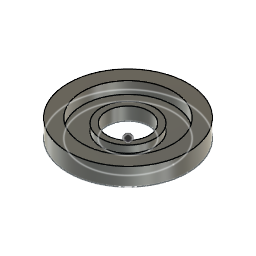
cap modified (Autodesk Fusion 360 design; units mm, degrees)
part number: 2025-11-25-15-10-51-182
Autodesk Fusion 360 part; units mm, degrees
sketch "Sketch1" plane through (0, 0, 0) normal (0, 0, 1) x (1, 0, 0)
  circle A0 centre (0, 0) radius 17.65
  circle A1 centre (0, 0) radius 38
  circle A2 centre (0, 0) radius 50
  dimension "d1" = 35.3
  dimension "d2" = 76
  dimension "d3" = 100
  constraint coincident A0.centre A1.centre
  measures "d1" diameter of A0
  measures "d2" diameter of A1
  measures "d3" diameter of A2
extrude "Extrude1" add sketch "Sketch1" along normal blind 5 contours A1
extrude "Extrude2" add sketch "Sketch1" along normal blind 15 contours A2
sketch "Sketch2" plane through (0, 0, 5) normal (0, 0, 1) x (-1, 0, 0)
  circle A0 centre (0, 0) radius 17.65
  circle A1 centre (0, 0) radius 38
  circle A2 centre (0, 0) radius 22.5
  dimension "d8" = 45
  constraint coincident A0.centre A1.centre
  measures "d8" diameter of A2
extrude "Extrude3" add sketch "Sketch2" along normal blind 6 contours A2
